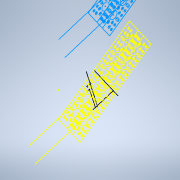
# Autodesk Inventor part: ring holder
Saved by Autodesk Inventor 2021 (Build 250183000, 183)
## iProperties
Created: 2021-03-22
Part Number: ring holder
Material: Generic
Document SubType Name: Modeling
Designer: deli
Density: 1 g/cm^3
Appearance: Default
Author: deli
Autodesk Inventor part; units mm, degrees
ref_plane "YZ Plane" through (0, 0, 0) normal (1, 0, 0) x (0, 1, 0)
ref_plane "XZ Plane" through (0, 0, 0) normal (0, 1, 0) x (-1, 0, 0)
ref_plane "XY Plane" through (0, 0, 0) normal (0, 0, 1) x (1, 0, 0)
sketch "Sketch1" plane through (0, 0, 0) normal (1, 0, 0) x (0, 1, 0)
  line L0 (64.4555, -41.9909) -> (61.5977, -32.9047)
  line L1 (138.014, 47.3051) -> (165.5457, 7.9858) projected
  line L2 (27.9282, -88.3751) -> (165.5457, 7.9858) projected
  line L3 (0.3965, -49.0558) -> (27.9282, -88.3751) projected
  line L4 (0.3965, -49.0558) -> (138.014, 47.3051) projected
  circle A0 centre (132.1202, 13.8796) radius 7 projected
  circle A1 centre (112.4606, 0.1137) radius 7 projected
  arc A2 (128.0668, 2.4092) -> (132.006, 1.7146) centre (130.0364, 2.0619) ccw projected
  line L5 (132.1252, 2.3905) -> (132.006, 1.7146) projected
  arc A3 (132.1252, 2.3905) -> (128.186, 3.085) centre (130.1556, 2.7377) ccw projected
  line L6 (128.0668, 2.4092) -> (128.186, 3.085) projected
  line L7 (120.5811, 8.2413) -> (121.7054, 9.0286) projected
  arc A4 (120.5811, 8.2413) -> (122.8754, 4.9647) centre (121.7282, 6.603) ccw projected
  line L8 (123.9997, 5.752) -> (122.8754, 4.9647) projected
  arc A5 (123.9997, 5.752) -> (121.7054, 9.0286) centre (122.8526, 7.3903) ccw projected
  arc A6 (120.6498, 17.933) -> (119.9552, 13.9937) centre (120.3025, 15.9634) ccw projected
  line L9 (120.6311, 13.8746) -> (119.9552, 13.9937) projected
  arc A7 (120.6311, 13.8746) -> (121.3257, 17.8138) centre (120.9784, 15.8442) ccw projected
  line L10 (120.6498, 17.933) -> (121.3257, 17.8138) projected
  arc A8 (143.5906, 9.8262) -> (144.2852, 13.7654) centre (143.9379, 11.7958) ccw projected
  line L11 (143.6093, 13.8846) -> (144.2852, 13.7654) projected
  arc A9 (143.6093, 13.8846) -> (142.9147, 9.9454) centre (143.262, 11.915) ccw projected
  line L12 (143.5906, 9.8262) -> (142.9147, 9.9454) projected
  line L13 (143.6594, 19.5178) -> (142.535, 18.7305) projected
  arc A10 (143.6594, 19.5178) -> (141.3651, 22.7944) centre (142.5122, 21.1561) ccw projected
  line L14 (140.2407, 22.0072) -> (141.3651, 22.7944) projected
  arc A11 (140.2407, 22.0072) -> (142.535, 18.7305) centre (141.3879, 20.3689) ccw projected
  line L15 (140.2478, 5.7591) -> (142.9357, 1.9203) projected
  arc A12 (140.2478, 5.7591) -> (136.9712, 3.4648) centre (138.6095, 4.6119) ccw projected
  line L16 (139.6591, -0.374) -> (136.9712, 3.4648) projected
  arc A13 (139.6591, -0.374) -> (142.9357, 1.9203) centre (141.2974, 0.7731) ccw projected
  circle A14 centre (134.7442, -3.8155) radius 2 projected
  circle A15 centre (128.191, -8.4041) radius 2 projected
  line L17 (120.5881, -8.0068) -> (123.2761, -11.8455) projected
  arc A16 (120.5881, -8.0068) -> (117.3115, -10.3011) centre (118.9498, -9.1539) ccw projected
  line L18 (119.9995, -14.1398) -> (117.3115, -10.3011) projected
  arc A17 (119.9995, -14.1398) -> (123.2761, -11.8455) centre (121.6378, -12.9927) ccw projected
  circle A18 centre (115.0846, -17.5813) radius 2 projected
  circle A19 centre (108.5314, -22.1699) radius 2 projected
  line L19 (100.9285, -21.7726) -> (103.6164, -25.6114) projected
  arc A20 (100.9285, -21.7726) -> (97.6519, -24.0669) centre (99.2902, -22.9197) ccw projected
  line L20 (100.3398, -27.9057) -> (97.6519, -24.0669) projected
  arc A21 (100.3398, -27.9057) -> (103.6164, -25.6114) centre (101.9781, -26.7585) ccw projected
  circle A22 centre (95.4249, -31.3471) radius 2 projected
  circle A23 centre (88.8717, -35.9357) radius 2 projected
  line L21 (81.2688, -35.5384) -> (83.9568, -39.3772) projected
  arc A24 (81.2688, -35.5384) -> (77.9922, -37.8327) centre (79.6305, -36.6856) ccw projected
  line L22 (80.6802, -41.6715) -> (77.9922, -37.8327) projected
  arc A25 (80.6802, -41.6715) -> (83.9568, -39.3772) centre (82.3185, -40.5244) ccw projected
  circle A26 centre (75.7653, -45.113) radius 2 projected
  circle A27 centre (69.2121, -49.7016) radius 2 projected
  line L23 (61.6092, -49.3043) -> (64.2971, -53.143) projected
  arc A28 (61.6092, -49.3043) -> (58.3326, -51.5986) centre (59.9709, -50.4514) ccw projected
  line L24 (61.0205, -55.4373) -> (58.3326, -51.5986) projected
  arc A29 (61.0205, -55.4373) -> (64.2971, -53.143) centre (62.6588, -54.2902) ccw projected
  circle A30 centre (56.1056, -58.8788) radius 2 projected
  circle A31 centre (49.5524, -63.4674) radius 2 projected
  line L25 (41.9495, -63.0701) -> (44.6375, -66.9089) projected
  arc A32 (41.9495, -63.0701) -> (38.6729, -65.3644) centre (40.3112, -64.2172) ccw projected
  line L26 (41.3609, -69.2032) -> (38.6729, -65.3644) projected
  arc A33 (41.3609, -69.2032) -> (44.6375, -66.9089) centre (42.9992, -68.056) ccw projected
  circle A34 centre (36.446, -72.6446) radius 2 projected
  circle A35 centre (29.8928, -77.2333) radius 2 projected
  line L27 (123.9926, 22.0001) -> (121.3047, 25.8389) projected
  arc A36 (123.9926, 22.0001) -> (127.2692, 24.2944) centre (125.6309, 23.1472) ccw projected
  line L28 (124.5813, 28.1332) -> (127.2692, 24.2944) projected
  arc A37 (124.5813, 28.1332) -> (121.3047, 25.8389) centre (122.943, 26.986) ccw projected
  circle A38 centre (116.3898, 22.3974) radius 2 projected
  circle A39 centre (109.8366, 17.8088) radius 2 projected
  line L29 (104.333, 8.2342) -> (101.645, 12.073) projected
  arc A40 (104.333, 8.2342) -> (107.6096, 10.5285) centre (105.9713, 9.3814) ccw projected
  line L30 (104.9216, 14.3673) -> (107.6096, 10.5285) projected
  arc A41 (104.9216, 14.3673) -> (101.645, 12.073) centre (103.2833, 13.2202) ccw projected
  circle A42 centre (96.7301, 8.6316) radius 2 projected
  circle A43 centre (90.1769, 4.043) radius 2 projected
  line L31 (84.6733, -5.5316) -> (81.9854, -1.6928) projected
  arc A44 (84.6733, -5.5316) -> (87.9499, -3.2373) centre (86.3116, -4.3844) ccw projected
  line L32 (85.262, 0.6015) -> (87.9499, -3.2373) projected
  arc A45 (85.262, 0.6015) -> (81.9854, -1.6928) centre (83.6237, -0.5457) ccw projected
  circle A46 centre (77.0705, -5.1343) radius 2 projected
  circle A47 centre (70.5173, -9.7229) radius 2 projected
  line L33 (65.0137, -19.2974) -> (62.3257, -15.4586) projected
  arc A48 (65.0137, -19.2974) -> (68.2903, -17.0031) centre (66.652, -18.1503) ccw projected
  line L34 (65.6023, -13.1643) -> (68.2903, -17.0031) projected
  arc A49 (65.6023, -13.1643) -> (62.3257, -15.4586) centre (63.964, -14.3115) ccw projected
  circle A50 centre (57.4108, -18.9001) radius 2 projected
  circle A51 centre (50.8576, -23.4887) radius 2 projected
  line L35 (45.354, -33.0633) -> (42.6661, -29.2245) projected
  arc A52 (45.354, -33.0633) -> (48.6306, -30.769) centre (46.9923, -31.9161) ccw projected
  line L36 (45.9427, -26.9302) -> (48.6306, -30.769) projected
  arc A53 (45.9427, -26.9302) -> (42.6661, -29.2245) centre (44.3044, -28.0773) ccw projected
  circle A54 centre (37.7512, -32.6659) radius 2 projected
  circle A55 centre (31.198, -37.2546) radius 2 projected
  line L37 (25.6944, -46.8291) -> (23.0064, -42.9903) projected
  arc A56 (25.6944, -46.8291) -> (28.971, -44.5348) centre (27.3327, -45.6819) ccw projected
  line L38 (26.283, -40.696) -> (28.971, -44.5348) projected
  arc A57 (26.283, -40.696) -> (23.0064, -42.9903) centre (24.6447, -41.8432) ccw projected
  circle A58 centre (18.0915, -46.4318) radius 2 projected
  circle A59 centre (11.5383, -51.0204) radius 2 projected
  arc A60 (25.6327, -72.7688) -> (26.3273, -68.8296) centre (25.98, -70.7992) ccw projected
  line L39 (25.6514, -68.7104) -> (26.3273, -68.8296) projected
  arc A61 (25.6514, -68.7104) -> (24.9568, -72.6497) centre (25.3041, -70.68) ccw projected
  line L40 (25.6327, -72.7688) -> (24.9568, -72.6497) projected
  arc A62 (18.2157, -57.245) -> (14.2765, -56.5504) centre (16.2461, -56.8977) ccw projected
  line L41 (14.1573, -57.2263) -> (14.2765, -56.5504) projected
  arc A63 (14.1573, -57.2263) -> (18.0965, -57.9209) centre (16.1269, -57.5736) ccw projected
  line L42 (18.2157, -57.245) -> (18.0965, -57.9209) projected
  arc A64 (147.7265, 16.175) -> (151.6657, 15.4804) centre (149.6961, 15.8277) ccw projected
  line L43 (151.7849, 16.1563) -> (151.6657, 15.4804) projected
  arc A65 (151.7849, 16.1563) -> (147.8456, 16.8509) centre (149.8153, 16.5036) ccw projected
  line L44 (147.7265, 16.175) -> (147.8456, 16.8509) projected
  arc A66 (140.3095, 31.6988) -> (139.6149, 27.7596) centre (139.9622, 29.7292) ccw projected
  line L45 (140.2907, 27.6404) -> (139.6149, 27.7596) projected
  arc A67 (140.2907, 27.6404) -> (140.9853, 31.5796) centre (140.638, 29.61) ccw projected
  line L46 (140.3095, 31.6988) -> (140.9853, 31.5796) projected
  circle A68 centre (129.4962, 31.5746) radius 2 projected
  circle A69 centre (147.8506, 5.3618) radius 2 projected
  circle A70 centre (154.4039, 9.9504) radius 2 projected
  circle A71 centre (136.0494, 36.1632) radius 2 projected
  arc A72 (45.2924, -59.003) -> (45.987, -55.0638) centre (45.6397, -57.0334) ccw projected
  line L47 (45.3111, -54.9446) -> (45.987, -55.0638) projected
  arc A73 (45.3111, -54.9446) -> (44.6165, -58.8838) centre (44.9638, -56.9142) ccw projected
  line L48 (45.2924, -59.003) -> (44.6165, -58.8838) projected
  arc A74 (64.952, -45.2372) -> (65.6466, -41.2979) centre (65.2993, -43.2675) ccw projected
  line L49 (64.9707, -41.1788) -> (65.6466, -41.2979) projected
  arc A75 (64.9707, -41.1788) -> (64.2761, -45.118) centre (64.6234, -43.1484) ccw projected
  line L50 (64.952, -45.2372) -> (64.2761, -45.118) projected
  arc A76 (84.6117, -31.4713) -> (85.3063, -27.5321) centre (84.959, -29.5017) ccw projected
  line L51 (84.6304, -27.4129) -> (85.3063, -27.5321) projected
  arc A77 (84.6304, -27.4129) -> (83.9358, -31.3521) centre (84.2831, -29.3825) ccw projected
  line L52 (84.6117, -31.4713) -> (83.9358, -31.3521) projected
  arc A78 (104.2713, -17.7055) -> (104.9659, -13.7663) centre (104.6186, -15.7359) ccw projected
  line L53 (104.29, -13.6471) -> (104.9659, -13.7663) projected
  arc A79 (104.29, -13.6471) -> (103.5954, -17.5863) centre (103.9427, -15.6167) ccw projected
  line L54 (104.2713, -17.7055) -> (103.5954, -17.5863) projected
  arc A80 (123.931, -3.9397) -> (124.6256, -0.0004) centre (124.2783, -1.97) ccw projected
  line L55 (123.9497, 0.1188) -> (124.6256, -0.0004) projected
  arc A81 (123.9497, 0.1188) -> (123.2551, -3.8205) centre (123.6024, -1.8509) ccw projected
  line L56 (123.931, -3.9397) -> (123.2551, -3.8205) projected
  arc A82 (22.3516, -50.8962) -> (21.657, -54.8354) centre (22.0043, -52.8658) ccw projected
  line L57 (22.3328, -54.9546) -> (21.657, -54.8354) projected
  arc A83 (22.3328, -54.9546) -> (23.0274, -51.0154) centre (22.6801, -52.985) ccw projected
  line L58 (22.3516, -50.8962) -> (23.0274, -51.0154) projected
  arc A84 (42.0112, -37.1304) -> (41.3166, -41.0696) centre (41.6639, -39.1) ccw projected
  line L59 (41.9925, -41.1888) -> (41.3166, -41.0696) projected
  arc A85 (41.9925, -41.1888) -> (42.6871, -37.2495) centre (42.3398, -39.2192) ccw projected
  line L60 (42.0112, -37.1304) -> (42.6871, -37.2495) projected
  arc A86 (61.6709, -23.3645) -> (60.9763, -27.3038) centre (61.3236, -25.3342) ccw projected
  line L61 (61.6521, -27.4229) -> (60.9763, -27.3038) projected
  arc A87 (61.6521, -27.4229) -> (62.3467, -23.4837) centre (61.9994, -25.4533) ccw projected
  line L62 (61.6709, -23.3645) -> (62.3467, -23.4837) projected
  arc A88 (81.3305, -9.5987) -> (80.6359, -13.5379) centre (80.9832, -11.5683) ccw projected
  line L63 (81.3118, -13.6571) -> (80.6359, -13.5379) projected
  arc A89 (81.3118, -13.6571) -> (82.0064, -9.7179) centre (81.6591, -11.6875) ccw projected
  line L64 (81.3305, -9.5987) -> (82.0064, -9.7179) projected
  arc A90 (100.9902, 4.1671) -> (100.2956, 0.2279) centre (100.6429, 2.1975) ccw projected
  line L65 (100.9714, 0.1087) -> (100.2956, 0.2279) projected
  arc A91 (100.9714, 0.1087) -> (101.666, 4.048) centre (101.3187, 2.0783) ccw projected
  line L66 (100.9902, 4.1671) -> (101.666, 4.048) projected
  arc A92 (22.2828, -60.5879) -> (24.5771, -63.8645) centre (23.43, -62.2262) ccw projected
  line L67 (25.7015, -63.0772) -> (24.5771, -63.8645) projected
  arc A93 (25.7015, -63.0772) -> (23.4072, -59.8006) centre (24.5543, -61.4389) ccw projected
  line L68 (22.2828, -60.5879) -> (23.4072, -59.8006) projected
  line L69 (41.9425, -46.822) -> (43.0668, -46.0347) projected
  arc A94 (41.9425, -46.822) -> (44.2368, -50.0986) centre (43.0896, -48.4603) ccw projected
  line L70 (45.3611, -49.3113) -> (44.2368, -50.0986) projected
  arc A95 (45.3611, -49.3113) -> (43.0668, -46.0347) centre (44.214, -47.673) ccw projected
  line L71 (61.6021, -33.0562) -> (62.7265, -32.2689) projected
  arc A96 (61.6021, -33.0562) -> (63.8964, -36.3328) centre (62.7493, -34.6945) ccw projected
  line L72 (65.0208, -35.5455) -> (63.8964, -36.3328) projected
  arc A97 (65.0208, -35.5455) -> (62.7265, -32.2689) centre (63.8736, -33.9072) ccw projected
  line L73 (81.2618, -19.2903) -> (82.3861, -18.5031) projected
  arc A98 (81.2618, -19.2903) -> (83.5561, -22.567) centre (82.4089, -20.9287) ccw projected
  line L74 (84.6804, -21.7797) -> (83.5561, -22.567) projected
  arc A99 (84.6804, -21.7797) -> (82.3861, -18.5031) centre (83.5333, -20.1414) ccw projected
  line L75 (100.9214, -5.5245) -> (102.0458, -4.7372) projected
  arc A100 (100.9214, -5.5245) -> (103.2157, -8.8011) centre (102.0686, -7.1628) ccw projected
  line L76 (104.3401, -8.0138) -> (103.2157, -8.8011) projected
  arc A101 (104.3401, -8.0138) -> (102.0458, -4.7372) centre (103.1929, -6.3755) ccw projected
  arc A102 (29.7686, -66.42) -> (33.7078, -67.1146) centre (31.7382, -66.7673) ccw projected
  line L77 (33.827, -66.4387) -> (33.7078, -67.1146) projected
  arc A103 (33.827, -66.4387) -> (29.8877, -65.7441) centre (31.8574, -66.0914) ccw projected
  line L78 (29.7686, -66.42) -> (29.8877, -65.7441) projected
  arc A104 (49.4282, -52.6542) -> (53.3675, -53.3488) centre (51.3978, -53.0015) ccw projected
  line L79 (53.4866, -52.6729) -> (53.3675, -53.3488) projected
  arc A105 (53.4866, -52.6729) -> (49.5474, -51.9783) centre (51.517, -52.3256) ccw projected
  line L80 (49.4282, -52.6542) -> (49.5474, -51.9783) projected
  arc A106 (69.0879, -38.8883) -> (73.0271, -39.5829) centre (71.0575, -39.2356) ccw projected
  line L81 (73.1463, -38.9071) -> (73.0271, -39.5829) projected
  arc A107 (73.1463, -38.9071) -> (69.207, -38.2125) centre (71.1767, -38.5598) ccw projected
  line L82 (69.0879, -38.8883) -> (69.207, -38.2125) projected
  arc A108 (88.7475, -25.1225) -> (92.6867, -25.8171) centre (90.7171, -25.4698) ccw projected
  line L83 (92.8059, -25.1412) -> (92.6867, -25.8171) projected
  arc A109 (92.8059, -25.1412) -> (88.8667, -24.4466) centre (90.8363, -24.7939) ccw projected
  line L84 (88.7475, -25.1225) -> (88.8667, -24.4466) projected
  arc A110 (108.4072, -11.3567) -> (112.3464, -12.0512) centre (110.3768, -11.704) ccw projected
  line L85 (112.4656, -11.3754) -> (112.3464, -12.0512) projected
  arc A111 (112.4656, -11.3754) -> (108.5263, -10.6808) centre (110.496, -11.0281) ccw projected
  line L86 (108.4072, -11.3567) -> (108.5263, -10.6808) projected
  arc A112 (37.8754, -43.4792) -> (33.9361, -42.7846) centre (35.9057, -43.1319) ccw projected
  line L87 (33.817, -43.4605) -> (33.9361, -42.7846) projected
  arc A113 (33.817, -43.4605) -> (37.7562, -44.1551) centre (35.7866, -43.8078) ccw projected
  line L88 (37.8754, -43.4792) -> (37.7562, -44.1551) projected
  arc A114 (57.535, -29.7134) -> (53.5958, -29.0188) centre (55.5654, -29.3661) ccw projected
  line L89 (53.4766, -29.6946) -> (53.5958, -29.0188) projected
  arc A115 (53.4766, -29.6946) -> (57.4158, -30.3892) centre (55.4462, -30.0419) ccw projected
  line L90 (57.535, -29.7134) -> (57.4158, -30.3892) projected
  arc A116 (77.1947, -15.9475) -> (73.2554, -15.2529) centre (75.225, -15.6002) ccw projected
  line L91 (73.1363, -15.9288) -> (73.2554, -15.2529) projected
  arc A117 (73.1363, -15.9288) -> (77.0755, -16.6234) centre (75.1059, -16.2761) ccw projected
  line L92 (77.1947, -15.9475) -> (77.0755, -16.6234) projected
  arc A118 (96.8543, -2.1817) -> (92.9151, -1.4871) centre (94.8847, -1.8344) ccw projected
  line L93 (92.7959, -2.163) -> (92.9151, -1.4871) projected
  arc A119 (92.7959, -2.163) -> (96.7351, -2.8576) centre (94.7655, -2.5103) ccw projected
  line L94 (96.8543, -2.1817) -> (96.7351, -2.8576) projected
  arc A120 (116.514, 11.5841) -> (112.5747, 12.2787) centre (114.5443, 11.9314) ccw projected
  line L95 (112.4556, 11.6029) -> (112.5747, 12.2787) projected
  arc A121 (112.4556, 11.6029) -> (116.3948, 10.9083) centre (114.4252, 11.2556) ccw projected
  line L96 (116.514, 11.5841) -> (116.3948, 10.9083) projected
  arc A122 (136.1736, 25.35) -> (132.2344, 26.0446) centre (134.204, 25.6973) ccw projected
  line L97 (132.1152, 25.3687) -> (132.2344, 26.0446) projected
  arc A123 (132.1152, 25.3687) -> (136.0544, 24.6741) centre (134.0848, 25.0214) ccw projected
  line L98 (136.1736, 25.35) -> (136.0544, 24.6741) projected
  circle A124 centre (33.822, -54.9496) radius 7 projected
  circle A125 centre (53.4816, -41.1838) radius 7 projected
  circle A126 centre (73.1413, -27.4179) radius 7 projected
  circle A127 centre (92.8009, -13.6521) radius 7 projected
  line L99 (67.0567, -66.1353) -> (-45.0063, -101.3808) projected
  line L100 (55.6257, -29.7905) -> (-56.4373, -65.036) projected
  line L101 (67.0567, -66.1353) -> (106.2659, -53.8034)
  line L102 (71.5998, -64.7064) -> (64.4555, -41.9909)
  line L103 (60.1688, -28.3616) -> (55.6257, -29.7905)
  line L104 (61.5977, -32.9047) -> (60.1688, -28.3616)
  line L105 (53.9774, 4.6561) -> (76.4528, -66.8041)
  line L106 (69.2053, -0.8754) -> (115.7634, -67.3672)
  circle A128 centre (63.964, -14.3115) radius 2
  point P0 (0, 0)
  point P1 (58.1515, -8.6153)
  point P2 (75.4156, -63.5063)
  dimension "d0" = 4
  constraints: 14 end point, 4 perpendicular, 4 point on line, 1 centre point, 1 coincident, 1 collinear, 1 concentric, 1 midpoint, 1 parallel, 3 other
  measures "d0" distance between parallel lines of L104 L105
extrude "Extrusion1" add sketch "Sketch1" along normal blind 146 contours L105 A27 A87 L4 L106 L73 A98 L74 L2 | L2 L106 L101 L105 | L105 A27 | L74 A98 L73 L106 | L105 A87 | L21 A25 L22 A24 | L33 A128 L34 A48 | L52 A77 L51 A76 | L82 A107 L81 A106 | L92 A117 L91 A116 | A126 picked at (71.0054, -49.1019)
body "Solid1"
